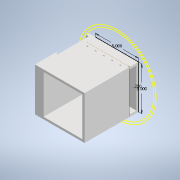
# Autodesk Inventor part: SqPot
Saved by Autodesk Inventor 2022 (Build 260153000, 153)
## iProperties
Created: 2021-11-11
Part Number: SqPot
Material: Generic
Document SubType Name: Modeling
Designer: aed0019
Density: 1 g/cm^3
Appearance: Default
Author: aed0019
Autodesk Inventor part; units mm, degrees
ref_plane "YZ Plane" through (0, 0, 0) normal (1, 0, 0) x (0, 1, 0)
ref_plane "XZ Plane" through (0, 0, 0) normal (0, 1, 0) x (-1, 0, 0)
ref_plane "XY Plane" through (0, 0, 0) normal (0, 0, 1) x (1, 0, 0)
sketch "Sketch1" plane through (0, 0, 0) normal (0, 0, 1) x (1, 0, 0)
  circle A0 centre (0, 0) radius 107.95 projected
  circle A1 centre (0, 0) radius 114.3 projected
  circle A2 centre (0, 0) radius 107.95 projected
  circle A3 centre (0, 0) radius 107.95 projected
  line L0 (-63.5, -63.5) -> (63.5, -63.5)
  line L1 (63.5, -63.5) -> (63.5, 63.5)
  line L2 (63.5, 63.5) -> (-63.5, 63.5)
  line L3 (-63.5, 63.5) -> (-63.5, -63.5)
  line L4 (-63.5, -63.5) -> (63.5, 63.5) construction
  line L5 (63.5, -63.5) -> (-63.5, 63.5) construction
  line L6 (57.15, 57.15) -> (57.15, -57.15)
  line L7 (57.15, -57.15) -> (-57.15, -57.15)
  line L8 (-57.15, -57.15) -> (-57.15, 57.15)
  line L9 (-57.15, 57.15) -> (57.15, 57.15)
  dimension "d0" = 127
  dimension "d1" = 127
  dimension "d2" = 6.35
  constraints: 20 end point, 4 parallel, 2 midpoint, 2 perpendicular, 1 horizontal, 3 other
  measures "d0" distance of L2.end L1.end
  measures "d1" distance of L1.end L0.end
  measures "d2" distance between parallel lines of L1 L6
extrude "Extrusion1" add sketch "Sketch1" along normal blind 6.35 contours L3 L2 L1 L0 | L6 L7 L8 L9
sketch "Sketch2" plane through (0, 0, 6.35) normal (0, 0, 1) x (1, 0, 0)
  line L0 (63.5, -63.5) -> (63.5, 63.5) projected
  line L1 (-63.5, 63.5) -> (63.5, 63.5)
  line L2 (63.5, 63.5) -> (63.5, -63.5)
  line L3 (63.5, -63.5) -> (-63.5, -63.5)
  line L4 (-63.5, -63.5) -> (-63.5, 63.5)
  line L5 (-63.5, 63.5) -> (63.5, -63.5) construction
  line L6 (63.5, 63.5) -> (-63.5, -63.5) construction
  line L7 (-57.15, -57.15) -> (57.15, -57.15)
  line L8 (57.15, -57.15) -> (57.15, 57.15)
  line L9 (57.15, 57.15) -> (-57.15, 57.15)
  line L10 (-57.15, 57.15) -> (-57.15, -57.15)
  point P0 (0, 0)
  dimension "d5" = 6.35
  constraints: 20 end point, 4 parallel, 2 midpoint, 2 perpendicular, 1 horizontal, 3 other
  measures "d5" distance between parallel lines of L3 L7
extrude "Extrusion2" add sketch "Sketch2" along normal blind 152.4
sketch "Sketch3" plane through (-63.5, -63.5, 0) normal (-1, 0, 0) x (0, 0, 1)
  line L0 (0, 127) -> (0, 0) projected
  line L1 (0, 0) -> (158.75, 0) projected
  line L2 (158.75, 127) -> (158.75, 0) projected
  line L3 (0, 127) -> (158.75, 127) projected
  point P0 (0, 63.5)
extrude "Extrusion3" add sketch "Sketch3" along normal blind 19.05
sketch "Sketch4" plane through (-82.55, -63.5, 0) normal (-1, 0, 0) x (0, 0, 1)
  line L0 (107.95, 6.35) -> (146.05, 6.35)
  line L1 (146.05, 6.35) -> (146.05, 120.65)
  line L2 (146.05, 120.65) -> (107.95, 120.65)
  line L3 (107.95, 120.65) -> (107.95, 6.35)
  line L4 (107.95, 6.35) -> (146.05, 120.65) construction
  line L5 (146.05, 6.35) -> (107.95, 120.65) construction
  line L6 (158.75, 127) -> (0, 127) projected
  line L7 (0, 0) -> (158.75, 0) projected
  line L8 (158.75, 0) -> (158.75, 127) projected
  point P0 (0, 63.5)
  point P1 (127, 63.5)
  dimension "d10" = 38.1
  dimension "d11" = 114.3
  dimension "d12" = 6.35
  dimension "d13" = 6.35
  dimension "d14" = 12.7
  constraints: 12 end point, 2 midpoint, 2 parallel, 1 horizontal, 1 perpendicular
  measures "d10" distance of L2.end L1.end
  measures "d11" distance of L1.end L0.end
  measures "d12" distance between parallel lines of L6 L2
  measures "d13" distance between parallel lines of L7 L0
  measures "d14" distance between parallel lines of L8 L1
extrude "Extrusion4" cut sketch "Sketch4" against normal blind 7.62
ref_plane "Work Plane1" through (0, 0, 25.4) normal (0, 0, 1) x (1, 0, 0)
sketch "Sketch6" plane through (0, 0, 25.4) normal (0, 0, 1) x (1, 0, 0)
  line L0 (-57.15, -57.15) -> (57.15, -57.15) projected
  line L1 (57.15, -57.15) -> (57.15, 57.15) projected
  line L2 (57.15, 57.15) -> (-57.15, 57.15) projected
  line L3 (-57.15, 57.15) -> (-57.15, -57.15) projected
  point P0 (0, 0)
extrude "Extrusion5" add sketch "Sketch6" along normal blind 6.35
sketch "Sketch7" plane through (63.5, 63.5, 158.75) normal (0, 1, 0) x (1, 0, 0)
  line L0 (-6.35, 133.35) -> (-120.65, 133.35) projected
  line L1 (-120.65, 127) -> (-6.35, 127) projected
  circle A0 centre (-19.05, 122.0738) radius 3.175
  circle A1 centre (-43.18, 122.0738) radius 3.175
  circle A2 centre (-67.31, 122.0738) radius 3.175
  circle A3 centre (-91.44, 122.0738) radius 3.175
  circle A4 centre (-115.57, 122.0738) radius 3.175
  line L2 (-15.875, 122.0738) -> (-22.225, 122.0738)
  line L3 (-40.005, 122.0738) -> (-46.355, 122.0738)
  line L4 (-64.135, 122.0738) -> (-70.485, 122.0738)
  line L5 (-88.265, 122.0738) -> (-94.615, 122.0738)
  line L6 (-112.395, 122.0738) -> (-118.745, 122.0738)
  point P0 (-63.5, 158.75)
  dimension "d20" = 6.35
  dimension "d21" = 12.7
  dimension "d24" = 24.13
  constraints: 10 end point, 10 point on circle, 5 centre point, 5 horizontal, 2 point on line, 8 other
  measures "d20" diameter of A0
  measures "d21" horizontal distance of L1.end A0.centre
  measures "d24" distance of A0.centre A1.centre
extrude "Extrusion6" cut sketch "Sketch7" against normal blind 127 contours L2 A0 | L3 A1 | L4 A2 | L5 A3 | L6 A4 picked at (-18.2578, 122.7756) picked at (-43.0524, 123.1244) picked at (-66.7088, 122.9448) picked at (-90.8388, 122.9448) picked at (-114.8476, 123.4366)
sketch "Sketch8" plane through (63.5, -63.5, 0) normal (1, 0, 0) x (0, 0, -1)
  line L0 (-6.35, 120.65) -> (-25.4, 120.65) projected
  line L1 (-158.75, 6.35) -> (-6.35, 6.35)
  line L2 (-6.35, 120.65) -> (-158.75, 120.65)
  line L3 (-6.35, 120.65) -> (-6.35, 6.35) projected
  line L4 (-6.35, 6.35) -> (-6.35, 120.65)
  line L5 (-28.575, 6.35) -> (-28.575, 120.65)
  point P0 (0, 63.5)
  point P1 (-25.4, 6.35)
  constraints: 8 end point, 1 horizontal, 1 parallel, 1 point on line, 1 vertical
extrude "Extrusion7" cut sketch "Sketch8" against normal blind 6.35
sketch "Sketch9" plane through (-57.15, 57.15, 6.35) normal (0, -1, 0) x (1, 0, 0)
  circle A0 centre (117.475, 19.05) radius 2.033
  line L0 (114.3, 19.05) -> (0, 19.05) projected
  line L1 (0, 0) -> (0, 19.05) projected
  line L2 (120.65, 0) -> (0, 0) projected
  line L3 (120.65, 22.225) -> (120.65, 0) projected
  line L4 (120.65, 22.225) -> (114.3, 22.225) projected
  line L5 (114.3, 22.225) -> (114.3, 19.05) projected
  point P0 (57.15, -6.35)
  dimension "d34" = 3.175
  dimension "d35" = 3.175
  constraints: 1 centre point
  measures "d34" distance from line of L4 A0.centre
  measures "d35" distance of L0.start A0.centre
extrude "Extrusion8" cut sketch "Sketch9" along normal mid plane 254 contours A0
sketch "Sketch10" plane through (0, 0, 0) normal (0, 0, -1) x (-1, 0, 0)
  line L0 (57.15, 57.15) -> (57.15, -57.15) projected
  line L1 (74.93, -57.15) -> (74.93, 57.15) projected
  line L2 (57.15, 57.15) -> (74.93, 57.15)
  line L3 (82.55, -57.15) -> (74.93, -57.15) projected
  line L4 (57.15, -57.15) -> (74.93, -57.15)
  line L5 (60.325, 57.15) -> (60.325, -57.15)
  point P0 (0, 0)
  dimension "d40" = 3.175
  constraints: 6 end point, 2 point on line, 1 horizontal, 1 perpendicular
  measures "d40" distance between parallel lines of L0 L5
extrude "Extrusion9" cut sketch "Sketch10" against normal blind 114.3 contours L2 L1 L4 L5
sketch "Sketch11" plane through (-82.55, -63.5, 0) normal (-1, 0, 0) x (0, 0, 1)
  line L0 (6.35, 120.65) -> (6.35, 6.35) projected
  line L1 (6.35, 120.65) -> (6.35, 6.35)
  line L2 (25.4, 120.65) -> (25.4, 6.35) projected
  line L3 (6.35, 6.35) -> (25.4, 6.35)
  line L4 (6.35, 120.65) -> (25.4, 120.65) projected
  line L5 (25.4, 120.65) -> (6.35, 120.65)
  point P0 (0, 63.5)
  constraints: 6 end point, 2 collinear, 1 perpendicular
extrude "Extrusion10" cut sketch "Sketch11" against normal blind 42.8625
sketch "Sketch12" plane through (-60.325, -57.15, 0) normal (-1, 0, 0) x (0, 0, 1)
  point P0 (0, 57.15)
sketch "Sketch13" plane through (-60.325, -57.15, 0) normal (-1, 0, 0) x (0, 0, 1)
  line L0 (0, 114.3) -> (6.35, 114.3) projected
  line L1 (6.35, 114.3) -> (0, 114.3)
  line L2 (0, 114.3) -> (0, -0.7007)
  line L3 (0, 120.65) -> (0, -6.35) projected
  line L4 (0, 0) -> (6.35, 0) projected
  line L5 (6.35, 0) -> (6.35, 114.3)
  point P0 (0, 57.15)
  constraints: 6 end point, 1 collinear, 1 perpendicular, 1 point on line
extrude "Extrusion11" add sketch "Sketch13" along normal blind 22.225
sketch "Sketch14" plane through (-82.55, -57.15, 25.4) normal (0, 0, -1) x (-1, 0, 0)
  line L0 (0, 114.3) -> (0, 0) projected
  line L1 (0, 114.3) -> (-7.62, 114.3) projected
  line L2 (0, 114.3) -> (-7.62, 114.3)
  line L3 (-7.62, 0) -> (-7.62, 114.3) projected
  line L4 (-7.62, 114.3) -> (-7.62, 0)
  line L5 (0, 0) -> (-7.62, 0) projected
  line L6 (-7.62, 0) -> (0, 0)
  line L7 (0, 0) -> (0, 114.3)
  point P0 (-82.55, 57.15)
  constraints: 8 end point, 2 collinear, 2 perpendicular
extrude "Extrusion12" add sketch "Sketch14" along normal blind 22.225
sketch "Sketch16" plane through (63.5, 63.5, 158.75) normal (0, 1, 0) x (1, 0, 0)
  line L0 (-138.43, 152.4) -> (-138.43, 50.8) projected
  line L1 (-138.43, 58.9187) -> (-142.4244, 58.9187)
  line L2 (-142.4244, 58.9187) -> (-142.4244, 64.1535)
  line L3 (-142.4244, 64.1535) -> (-146.05, 64.1535)
  line L4 (-146.05, 158.75) -> (-146.05, 0) projected
  line L5 (-146.05, 150.6067) -> (-137.3483, 150.6067)
  line L6 (-137.3483, 150.6067) -> (-137.3483, 58.9187)
  line L7 (-137.3483, 58.9187) -> (-138.43, 58.9187)
  point P0 (-63.5, 158.75)
  point P1 (-138.43, 150.6067)
  constraints: 12 end point, 4 perpendicular, 3 point on line, 2 horizontal
extrude "Extrusion13" cut sketch "Sketch16" against normal blind 122.2375 contours L0 L1 L2 L3 L4 L5
sketch "Sketch17" plane through (63.5, 63.5, 158.75) normal (0, 1, 0) x (1, 0, 0)
  line L0 (-138.43, 150.6067) -> (-138.43, 154.3098)
  line L1 (-138.43, 154.3098) -> (-141.7479, 154.3098)
  line L2 (-141.7479, 154.3098) -> (-141.7479, 150.6067)
  line L3 (-146.05, 150.6067) -> (-138.43, 150.6067) projected
  point P0 (-63.5, 158.75)
  constraints: 6 end point, 2 vertical, 1 perpendicular, 1 point on line
extrude "Extrusion14" cut sketch "Sketch17" against normal blind 122.2375
body "Solid1"
